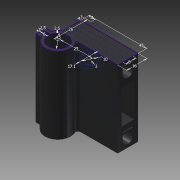
# Autodesk Inventor part: X_base
Saved by Autodesk Inventor 2013 (Build 170138000, 138)
## iProperties
Created: 2014-01-22
Part Number: X_base
Material: Generic
Document SubType Name: Modeling
Designer: Masta
Density: 1 g/cm^3
Author: Masta
Autodesk Inventor part; units mm, degrees
ref_plane "YZ Plane" through (0, 0, 0) normal (1, 0, 0) x (0, 1, 0)
ref_plane "XZ Plane" through (0, 0, 0) normal (0, 1, 0) x (-1, 0, 0)
sketch "Sketch2" plane through (0, 0, 0) normal (0, 0, 1) x (1, 0, 0)
  line L0 (0, 0) -> (25, 0) construction
  circle A0 centre (0, 0) radius 7.5 construction
  line L1 (15.1273, 0) -> (20.0637, 8.55) construction
  line L2 (20.0637, 8.55) -> (29.9363, 8.55) construction
  line L3 (29.9363, 8.55) -> (34.8727, 0) construction
  line L4 (34.8727, 0) -> (29.9363, -8.55) construction
  line L5 (29.9363, -8.55) -> (20.0637, -8.55) construction
  line L6 (20.0637, -8.55) -> (15.1273, 0) construction
  line L7 (0, 0) -> (0, 26) construction
  line L8 (0, 26) -> (25, 26) construction
  line L9 (-7.3485, 1.5) -> (-13.3485, 1.5)
  line L10 (-13.3485, 1.5) -> (-13.3485, -1.5) construction
  line L11 (-13.3485, -1.5) -> (-7.3485, -1.5)
  line L12 (-13.3485, -1.5) -> (-13.3485, -4)
  line L13 (-13.3485, 1.5) -> (-13.3485, 4)
  line L14 (-5, 23) -> (-5, 8.6603)
  arc A1 (-5, 8.6603) -> (-9.1652, 4) centre (0, 0) ccw
  line L15 (-13.3485, 4) -> (-9.1652, 4)
  line L16 (-13.3485, -4) -> (-9.1652, -4)
  arc A2 (-9.1652, 4) -> (-9.1652, -4) centre (0, 0) ccw construction
  arc A3 (-9.1652, -4) -> (7.1414, 7) centre (0, 0) ccw
  line L17 (-5, 23) -> (40, 23)
  arc A4 (-7.3485, -1.5) -> (-7.3485, 1.5) centre (0, 0) ccw
  circle A5 centre (25, 0) radius 5 construction
  circle A6 centre (25, 0) radius 6 construction
  line L18 (40, 23) -> (40, 7)
  line L19 (40, 7) -> (7.1414, 7)
  line L20 (40, 15) -> (-5, 15) construction
  line L21 (40, 19) -> (-5, 19) construction
  line L22 (-5, 11) -> (40, 11) construction
  dimension "d32" = 25
  dimension "d33" = 15
  dimension "d34" = 17.1
  dimension "d35" = 26
  dimension "d36" = 6
  dimension "d37" = 2.5
  dimension "d38" = 3
  dimension "d39" = 2.5
  dimension "d40" = 3
  dimension "d41" = 10
  dimension "d42" = 1
  dimension "d43" = 16
  dimension "d44" = 8
  dimension "d45" = 5
  dimension "d46" = 45
  constraints: 46 end point, 10 perpendicular, 10 point on circle, 8 coincident, 7 centre point, 6 point on line, 5 parallel, 2 collinear, 1 concentric, 1 horizontal, 1 midpoint, 15 other
  measures "d32" distance of L0.start L0.end
  measures "d33" diameter of A0
  measures "d34" distance between parallel lines of L5 L2
  measures "d35" distance of L7.start L7.end
  measures "d36" distance of L10.end L11.end
  measures "d37" distance of L9.end L13.end
  measures "d38" distance of L9.end L10.end
  measures "d39" radial gap between concentric circles of A1 A0
  measures "d40" distance between parallel lines of L8 L17
  measures "d41" diameter of A5
  measures "d42" radial gap between concentric circles of A6 A5
  measures "d43" distance between parallel lines of L19 L17
  measures "d44" distance between parallel lines of L22 L21
  measures "d45" distance between parallel lines of L7 L14
  measures "d46" distance between parallel lines of L18 L14
extrude "Extrusion6" add sketch "Sketch2" against normal blind 60
fillet "Fillet1" radius 2 2 edges at (7.1414, 7, -30) (-5, 8.6603, -30)
ref_plane "Work Plane1" through (0, 0, -30) normal (0, 0, 1) x (1, 0, 0)
sketch "Sketch4" plane through (40, 7, 0) normal (1, 0, 0) x (0, 0, -1)
  line L0 (0, 16) -> (0, 0) projected
  line L1 (60, 16) -> (60, 0) projected
  line L2 (0, 8) -> (60, 8) construction
  circle A0 centre (8.5, 8) radius 4
  line L3 (4.5, 4) -> (8.5, 4)
  line L4 (8.5, 4) -> (8.5, 12)
  line L5 (8.5, 12) -> (4.5, 12)
  line L6 (4.5, 12) -> (4.5, 4)
  line L7 (4.5, 4) -> (8.5, 12) construction
  line L8 (8.5, 4) -> (4.5, 12) construction
  line L9 (3.3, 4) -> (2.4, 4)
  line L10 (2.4, 4) -> (2.4, 12)
  line L11 (2.4, 12) -> (3.3, 12)
  line L12 (3.3, 12) -> (3.3, 4)
  line L13 (3.3, 4) -> (2.4, 12) construction
  line L14 (2.4, 4) -> (3.3, 12) construction
  circle A1 centre (53.5, 8) radius 4
  line L15 (49.5, 4) -> (53.5, 4)
  line L16 (53.5, 4) -> (53.5, 12)
  line L17 (53.5, 12) -> (49.5, 12)
  line L18 (49.5, 12) -> (49.5, 4)
  line L19 (49.5, 4) -> (53.5, 12) construction
  line L20 (53.5, 4) -> (49.5, 12) construction
  line L21 (48.3, 4) -> (47.4, 4)
  line L22 (47.4, 4) -> (47.4, 12)
  line L23 (47.4, 12) -> (48.3, 12)
  line L24 (48.3, 12) -> (48.3, 4)
  line L25 (48.3, 4) -> (47.4, 12) construction
  line L26 (47.4, 4) -> (48.3, 12) construction
  line L27 (43.4, 3) -> (16.6, 3)
  line L28 (16.6, 3) -> (16.6, 13)
  line L29 (16.6, 13) -> (43.4, 13)
  line L30 (43.4, 13) -> (43.4, 3)
  line L31 (43.4, 3) -> (16.6, 13) construction
  line L32 (16.6, 3) -> (43.4, 13) construction
  line L33 (47.4, 8) -> (43.4, 8) construction
  line L34 (12.5, 8) -> (16.6, 8) construction
  point P0 (0, -7)
  point P1 (6.5, 8)
  point P2 (2.85, 8)
  point P3 (51.5, 8)
  point P4 (47.85, 8)
  point P5 (30, 8)
  dimension "d52" = 8
  dimension "d53" = 0.9
  dimension "d54" = 1.2
  dimension "d55" = 2.4
  dimension "d58" = 45
  dimension "d63" = 10
  dimension "d65" = 4
  constraints: 66 end point, 18 midpoint, 6 parallel, 5 horizontal, 4 point on line, 3 perpendicular, 1 centre point, 1 collinear, 1 horizontal alignment, 1 line through centre, 1 vertical, 25 other
  measures "d53" distance of L10.end L11.end
  measures "d54" distance between parallel lines of L6 L12
  measures "d55" distance between parallel lines of L0 L10
  measures "d58" distance of L9.end L21.end
  measures "d63" distance of L27.end L28.end
  measures "d65" distance between parallel lines of L22 L30
extrude "Extrusion7" cut sketch "Sketch4" against normal up to next
body "Solid2"
